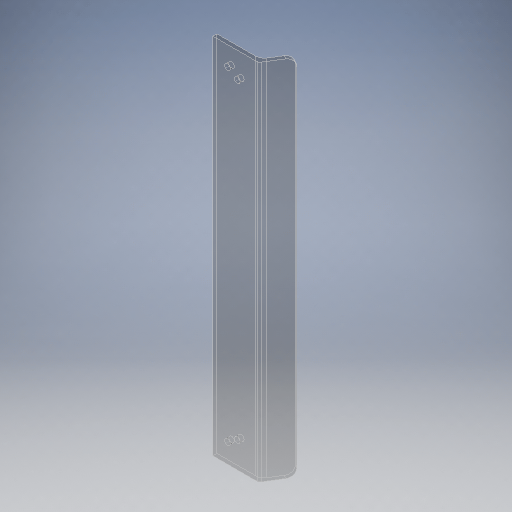
# Autodesk Inventor part: PolyIntakeTop
Saved by Autodesk Inventor 2026.1 (Build 301233000, 233)
## iProperties
Created: 2025-09-29
Part Number: PolyIntakeTop
Material: Polycarbonate, Smoke
Document SubType Name: Modeling
Designer: Teddy
Density: 1.2 g/cm^3
Appearance: Polycarbonate - Smoked
Author: Teddy
Autodesk Inventor part; units mm, degrees
ref_plane "YZ Plane" through (0, 0, 0) normal (1, 0, 0) x (0, 1, 0)
ref_plane "XZ Plane" through (0, 0, 0) normal (0, 1, 0) x (-1, 0, 0)
ref_plane "Work Plane1" through (0, 0, 0) normal (0, 0, 1) x (1, 0, 0)
sketch "Sketch1" plane through (0, 0, 0) normal (0, 0, 1) x (1, 0, 0)
  circle A0 centre (11.43, 2.54) radius 2.286 projected
  circle A1 centre (19.05, 7.62) radius 2.286 projected
  circle A2 centre (19.05, 252.2398) radius 2.286 projected
  circle A3 centre (11.43, 257.3198) radius 2.286 projected
  line L0 (22.225, -12.7) -> (-22.225, -12.7) projected
  line L1 (22.225, 272.5598) -> (-22.225, 272.5598) projected
  line L2 (34.925, -12.7) -> (-22.225, -12.7)
  line L3 (-22.225, -12.7) -> (-22.225, 272.5598) construction
  line L4 (-22.225, 272.5598) -> (34.925, 272.5598)
  line L5 (34.925, 272.5598) -> (34.925, -12.7)
  line L6 (0, 272.5598) -> (0, -12.7)
  point P0 (0, 0)
  point P1 (-22.225, -12.7)
  point P2 (0, -12.7)
  point P3 (0, -12.7)
  dimension "d0" = 57.15
  dimension "d9" = 34.925
  constraints: 10 end point, 2 parallel, 2 perpendicular, 2 point on line, 1 horizontal, 1 midpoint, 1 vertical alignment
  measures "d0" distance between parallel lines of L3 L5
  measures "d9" distance between parallel lines of L5 L6
extrude "Extrusion1" add sketch "Sketch1" along normal blind 3.175
sketch "Sketch2" plane through (-22.225, 272.5598, 0) normal (0, 1, 0) x (1, 0, 0)
  line L0 (69.8754, 18.7905) -> (57.15, -1.5875) construction
  line L1 (57.15, 0) -> (57.15, -3.175) projected
  line L2 (66.9043, 17.0297) -> (55.5406, -1.1676)
  line L3 (69.5973, 15.348) -> (58.7765, -1.98)
  arc A0 (57.15, -3.175) -> (58.7765, -1.98) centre (56.4627, -0.5351) ccw
  line L4 (57.15, -3.175) -> (55.5406, -1.1676)
  line L5 (69.5973, 15.348) -> (66.9043, 17.0297)
  point P0 (22.225, 0)
  dimension "d4" = 1.5875
  dimension "d5" = 1.5875
  constraints: 10 end point, 2 parallel, 2 point on circle, 1 centre point, 1 midpoint, 1 perpendicular, 1 tangent
  measures "d4" distance between parallel lines of L0 L2
  measures "d5" distance between parallel lines of L0 L3
extrude "Extrusion2" add sketch "Sketch2" against normal up to surface (285.2598 mm away)
fillet "Fillet1" radius 6.35 3 edges at (46.0258, 272.5598, -16.1889) (34.0447, 129.9299, 0) (46.0258, -12.7, -16.1889)
body "Solid1"
